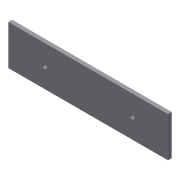
# Autodesk Inventor part: Lower Motor Mount
Saved by Autodesk Inventor 2015 (Build 190159000, 159)
## iProperties
Created: 2015-01-24
Part Number: Lower Motor Mount
Material: Generic
Document SubType Name: Modeling
Designer: Peter
Density: 1 g/cm^3
Appearance: Default
Author: Peter
Autodesk Inventor part; units mm, degrees
ref_plane "YZ Plane" through (0, 0, 0) normal (1, 0, 0) x (0, 1, 0)
ref_plane "XZ Plane" through (0, 0, 0) normal (0, 1, 0) x (-1, 0, 0)
ref_plane "XY Plane" through (0, 0, 0) normal (0, 0, 1) x (1, 0, 0)
sketch "Sketch1" plane through (0, 0, 0) normal (0, 0, 1) x (1, 0, 0)
  line L0 (0, 0) -> (203.2, 0)
  line L1 (203.2, 0) -> (203.2, 50.8)
  line L2 (203.2, 50.8) -> (0, 50.8)
  line L3 (0, 50.8) -> (0, 0)
  dimension "d0" = 203.2
  dimension "d1" = 50.8
  constraints: 8 end point, 2 parallel, 1 horizontal, 1 perpendicular
  measures "d0" distance of L2.end L1.end
  measures "d1" distance of L1.end L0.end
extrude "Extrusion1" add sketch "Sketch1" along normal blind 4.826
sketch "Sketch3" plane through (0, 0, 4.826) normal (0, 0, 1) x (1, 0, 0)
  line L0 (0, 0) -> (203.2, 0) projected
  line L1 (203.2, 50.8) -> (0, 50.8) projected
  circle A0 centre (46.0121, 35.4232) radius 4.2545 projected
  circle A1 centre (157.1371, 35.4232) radius 4.2545 projected
  line L2 (46.0121, 0) -> (46.0121, 50.8) construction
  line L3 (157.1371, 0) -> (157.1371, 50.8) construction
  circle A2 centre (46.0121, 25.4) radius 3.175
  circle A3 centre (157.1371, 25.4) radius 3.175
  dimension "d11" = 6.35
  dimension "d12" = 6.35
  constraints: 4 end point, 4 point on line, 2 centre point, 2 coincident, 2 midpoint, 1 parallel, 1 perpendicular
  measures "d11" diameter of A2
  measures "d12" diameter of A3
extrude "Extrusion2" cut sketch "Sketch3" against normal blind 6.35 contours A2 | A3
equation "\"d13\" = d12"
body "Solid1"
